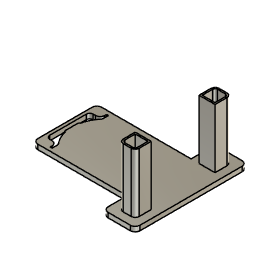
daq_cclamp_3t v2 (Autodesk Fusion 360 design; units mm, degrees)
Autodesk Fusion 360 part; units mm, degrees
sketch "Sketch3" plane through (0, 0, 31.5) normal (0, 0, 1) x (-1, 0, 0)
  arc A0 (-4.334986, -24.725) -> (-4.847966, -25.138298) centre (-4.334986, -25.25) ccw
  line L0 (-4.334986, -24.725) -> (-3.955328, -24.725)
  line L1 (-3.955328, -24.725) -> (-3.955328, -15.275)
  line L2 (-3.955328, -15.275) -> (-4.334986, -15.275)
  arc A1 (-4.847966, -14.861702) -> (-4.334986, -15.275) centre (-4.334986, -14.75) ccw
  arc A2 (-4.847966, -14.861702) -> (-5.656416, -12.00609) centre (-28.445008, -20) ccw
  arc A3 (-5.656416, -12.00609) -> (-9.099786, -6.138625) centre (-23.872376, -18.752159) ccw
  arc A4 (-9.60275, -4.775) -> (-9.099786, -6.138625) centre (-7.50275, -4.775) ccw
  line L3 (-9.60275, -4.775) -> (-9.60275, -1.625)
  line L4 (-9.60275, -1.625) -> (-8.55275, -1.625)
  line L5 (-8.55275, -1.625) -> (-8.55275, -2.675)
  arc A5 (-8.55275, -2.675) -> (-5.40275, -5.825) centre (-5.40275, -2.675) ccw
  line L6 (-5.40275, -5.825) -> (-3.82775, -5.825)
  arc A6 (-1.72775, -7.925) -> (-3.82775, -5.825) centre (-3.82775, -7.925) ccw
  line L7 (-1.72775, -7.925) -> (-1.72775, -32.075)
  arc A7 (-3.82775, -34.175) -> (-1.72775, -32.075) centre (-3.82775, -32.075) ccw
  line L8 (-3.82775, -34.175) -> (-5.40275, -34.175)
  arc A8 (-5.40275, -34.175) -> (-8.55275, -37.325) centre (-5.40275, -37.325) ccw
  line L9 (-8.55275, -37.325) -> (-8.55275, -38.375)
  line L10 (-8.55275, -38.375) -> (-9.60275, -38.375)
  line L11 (-9.60275, -38.375) -> (-9.60275, -35.225)
  arc A9 (-9.099786, -33.861375) -> (-9.60275, -35.225) centre (-7.50275, -35.225) ccw
  arc A10 (-9.099786, -33.861375) -> (-5.656416, -27.99391) centre (-23.872376, -21.247841) ccw
  arc A11 (-5.656416, -27.99391) -> (-4.847966, -25.138298) centre (-28.445008, -20) ccw
  arc A12 (-3, -40) -> (0, -37) centre (-3, -37) ccw
  line L12 (0, -37) -> (0, -3)
  arc A13 (0, -3) -> (-3, 0) centre (-3, -3) ccw
  line L13 (-3, 0) -> (-11, 0)
  line L14 (-11, 0) -> (-11, -40)
  line L15 (-11, -40) -> (-3, -40)
  line L16 (-62, -55) -> (-76, -55)
  line L17 (-79, -52) -> (-79, 12)
  line L18 (-76, 15) -> (-62, 15)
  line L19 (-59, 12) -> (-59, -52)
  line L20 (-11, -40) -> (-59, -40)
  line L21 (-59, -40) -> (-59, 0)
  line L22 (-59, 0) -> (-11, 0)
  line L23 (-11, 0) -> (-11, -40)
  arc A14 (-79, -52) -> (-76, -55) centre (-76, -52) ccw
  arc A15 (-76, 15) -> (-79, 12) centre (-76, 12) ccw
  arc A16 (-59, 12) -> (-62, 15) centre (-62, 12) ccw
  arc A17 (-62, -55) -> (-59, -52) centre (-62, -52) ccw
  arc A18 (-9.054822, -33.201309) -> (-9.533835, -34.5) centre (-7.533835, -34.5) ccw
  arc A19 (-9.130871, -33.136375) -> (-5.869498, -27.57933) centre (-23.123955, -21.18842) ccw
  line L24 (-8.433835, -3.5) -> (-8.433835, -2.4)
  arc A20 (-9.130871, -33.136375) -> (-9.633835, -34.5) centre (-7.533835, -34.5) ccw
  arc A21 (-8.433835, -3.5) -> (-5.533835, -6.4) centre (-5.533835, -3.5) ccw
  arc A22 (-5.717538, -12.54527) -> (-5.775422, -12.386752) centre (-23.123955, -18.81158) ccw
  line L25 (-4.033835, -6.5) -> (-5.533835, -6.5)
  arc A23 (-5.005469, -15.106383) -> (-5.775422, -12.386752) centre (-27.478842, -20) ccw
  line L26 (-9.633835, -2.4) -> (-9.633835, -5.5)
  arc A24 (-5.775422, -27.613248) -> (-5.717538, -27.45473) centre (-23.123955, -21.18842) ccw
  line L27 (-9.533835, -34.5) -> (-9.533835, -37.5)
  arc A25 (-5.533835, -33.5) -> (-8.533835, -36.5) centre (-5.533835, -36.5) ccw
  line L28 (-5.533835, -33.6) -> (-4.033835, -33.6)
  arc A26 (-9.054822, -33.201309) -> (-5.775422, -27.613248) centre (-23.123955, -21.18842) ccw
  arc A27 (-4.516917, -24.4) -> (-5.103179, -24.87234) centre (-4.516917, -25) ccw
  arc A28 (-5.533835, -33.6) -> (-8.433835, -36.5) centre (-5.533835, -36.5) ccw
  arc A29 (-5.005469, -15.106383) -> (-4.516917, -15.5) centre (-4.516917, -15) ccw
  line L29 (-9.533835, -2.5) -> (-9.533835, -5.5)
  arc A30 (-4.033835, -33.6) -> (-1.933835, -31.5) centre (-4.033835, -31.5) ccw
  line L30 (-4.255338, -24.4) -> (-4.516917, -24.4)
  line L31 (-4.516917, -15.5) -> (-4.155338, -15.5)
  arc A31 (-5.775422, -12.386752) -> (-9.054822, -6.798691) centre (-23.123955, -18.81158) ccw
  line L32 (-8.433835, -37.6) -> (-8.433835, -36.5)
  line L33 (-9.633835, -37.6) -> (-8.433835, -37.6)
  arc A32 (-4.516917, -24.5) -> (-5.005469, -24.893617) centre (-4.516917, -25) ccw
  arc A33 (-5.869498, -27.57933) -> (-5.103179, -24.87234) centre (-27.478842, -20) ccw
  arc A34 (-9.533835, -5.5) -> (-9.054822, -6.798691) centre (-7.533835, -5.5) ccw
  line L34 (-5.717538, -27.45473) -> (-5.838432, -27.790548)
  line L35 (-8.433835, -2.4) -> (-9.633835, -2.4)
  arc A35 (-8.533835, -3.5) -> (-5.533835, -6.5) centre (-5.533835, -3.5) ccw
  line L36 (-4.516917, -15.6) -> (-4.255338, -15.6)
  line L37 (-5.838432, -12.209452) -> (-5.717538, -12.54527)
  line L38 (-8.533835, -2.5) -> (-9.533835, -2.5)
  line L39 (-4.155338, -24.5) -> (-4.516917, -24.5)
  line L40 (-9.533835, -37.5) -> (-8.533835, -37.5)
  arc A36 (-2.033835, -8.5) -> (-4.033835, -6.5) centre (-4.033835, -8.5) ccw
  arc A37 (-5.869498, -12.42067) -> (-9.130871, -6.863625) centre (-23.123955, -18.81158) ccw
  arc A38 (-5.775422, -12.386752) -> (-5.838432, -12.209452) centre (-27.478842, -20) ccw
  arc A39 (-5.838432, -27.790548) -> (-5.775422, -27.613248) centre (-27.478842, -20) ccw
  arc A40 (-1.933835, -8.5) -> (-4.033835, -6.4) centre (-4.033835, -8.5) ccw
  line L41 (-0.033835, -40) -> (-0.033835, 0)
  line L42 (-11.033835, 0) -> (-11.033835, -40)
  line L43 (-0.033835, 0) -> (-11.033835, 0)
  line L44 (-11.033835, -40) -> (-0.033835, -40)
  arc A41 (-5.775422, -27.613248) -> (-5.005469, -24.893617) centre (-27.478842, -20) ccw
  line L45 (-4.155338, -15.5) -> (-4.155338, -24.5)
  line L46 (-1.933835, -31.5) -> (-1.933835, -8.5)
  line L47 (-2.033835, -31.5) -> (-2.033835, -8.5)
  line L48 (-4.255338, -15.6) -> (-4.255338, -24.4)
  arc A42 (-4.033835, -33.5) -> (-2.033835, -31.5) centre (-4.033835, -31.5) ccw
  line L49 (-4.033835, -6.4) -> (-5.533835, -6.4)
  line L50 (-8.533835, -3.5) -> (-8.533835, -2.5)
  arc A43 (-5.103179, -15.12766) -> (-4.516917, -15.6) centre (-4.516917, -15) ccw
  line L51 (-5.533835, -33.5) -> (-4.033835, -33.5)
  line L52 (-8.533835, -37.5) -> (-8.533835, -36.5)
  arc A44 (-9.633835, -5.5) -> (-9.130871, -6.863625) centre (-7.533835, -5.5) ccw
  line L53 (-9.633835, -34.5) -> (-9.633835, -37.6)
  arc A45 (-5.103179, -15.12766) -> (-5.869498, -12.42067) centre (-27.478842, -20) ccw
  point P0 (-59, -55)
  point P1 (-79, -55)
  point P2 (-59, 15)
  point P3 (-0.033835, 0)
  point P4 (-1.761584, -20)
  dimension "d17" = 20
  dimension "d18" = 70
  dimension "d19" = 48
  dimension "d20" = 40
  dimension "d21" = 3
  dimension "d61" = 0.1
  dimension "d62" = 11
  dimension "d63" = 40
  constraint horizontal L16
  constraint vertical L17
  constraint horizontal L18
  constraint vertical L19
  constraint horizontal L20
  constraint vertical L21
  constraint horizontal L22
  constraint vertical L23
  constraint coincident L14.end L15.start
  constraint coincident P1 L16
  constraint coincident P1 L17
  constraint tangent L16 A14
  constraint tangent L17 A14
  constraint tangent L17 A15
  constraint tangent L18 A15
  constraint equal A14 A15
  constraint coincident L19 L21
  constraint coincident P2 L18
  constraint coincident P2 L19
  constraint tangent L18 A16
  constraint tangent L19 A16
  constraint equal A14 A16
  constraint coincident P0 L16
  constraint coincident P0 L19
  constraint tangent L16 A17
  constraint tangent L19 A17
  constraint equal A14 A17
  measures "d17" distance of P0 P1
  measures "d18" distance of P0 P2
  measures "d19" distance of L14.end L20.end
  measures "d20" distance of L14.end L13.end
  measures "d21" radius of A14
extrude "Extrude3" add sketch "Sketch3" along normal blind 3 contours A22 L37 A38 | A24 L34 A39 | L9 L10 L11 L33 | A5 L6 A6 L7 A7 L8 A8 A21 L28 A28 A30 A40 L46 L49 | L3 L4 L5 L35 | A12 A13 L13 L14 L15 L23 L41 L43 L44 | A12 L12 A13 L41 | L14 L20 L22 L23 L42 L43 L44 | L19 L20 L21 L22 L42 | L16 L17 L18 L19 L21 A14 A15 A16 A17 picked at (-5.775884, -12.384627) picked at (-5.775884, -27.615373) picked at (-8.90275, -38.116667) picked at (-4.421445, -33.983333) picked at (-9.25275, -1.883333) picked at (-7.788307, -18.375887) picked at (-0.022556, -14.333333) picked at (-11.011278, -26.666667) picked at (-27.022556, -26.666667) picked at (-72.333333, -26.666667) makes body 1 at (42.482617, 24.545325, 34.5) makes body 2 at (5.798134, 12.321391, 33.5) makes body 3 at (5.757836, 27.566669, 33.5)
sketch "Sketch6" plane through (0, 0, 34.5) normal (0, 0, 1) x (-1, 0, 0)
  arc A0 (-79, -52) -> (-76, -55) centre (-76, -52) ccw
  line L0 (-76, -55) -> (-62, -55)
  arc A1 (-62, -55) -> (-59, -52) centre (-62, -52) ccw
  line L1 (-59, -52) -> (-59, -40)
  line L2 (-59, -40) -> (-3, -40)
  arc A2 (-3, -40) -> (0, -37) centre (-3, -37) ccw
  line L3 (0, -37) -> (0, -3)
  arc A3 (0, -3) -> (-3, 0) centre (-3, -3) ccw
  line L4 (-3, 0) -> (-59, 0)
  line L5 (-59, 0) -> (-59, 12)
  arc A4 (-59, 12) -> (-62, 15) centre (-62, 12) ccw
  line L6 (-62, 15) -> (-76, 15)
  arc A5 (-76, 15) -> (-79, 12) centre (-76, 12) ccw
  line L7 (-79, 12) -> (-79, -52)
  line L8 (-66.5, -50) -> (-71.5, -50)
  line L9 (-74, -47.5) -> (-74, -40)
  line L10 (-74, -40) -> (-64, -40)
  line L11 (-64, -40) -> (-64, -47.5)
  line L12 (-64, 0) -> (-74, 0)
  line L13 (-74, 0) -> (-74, 7.5)
  line L14 (-71.5, 10) -> (-66.5, 10)
  line L15 (-64, 7.5) -> (-64, 0)
  arc A6 (-66.5, -50) -> (-64, -47.5) centre (-66.5, -47.5) ccw
  arc A7 (-74, -47.5) -> (-71.5, -50) centre (-71.5, -47.5) ccw
  arc A8 (-71.5, 10) -> (-74, 7.5) centre (-71.5, 7.5) ccw
  arc A9 (-64, 7.5) -> (-66.5, 10) centre (-66.5, 7.5) ccw
  line L16 (-4.255338, -15.6) -> (-4.516917, -15.6)
  arc A10 (-5.103179, -15.12766) -> (-4.516917, -15.6) centre (-4.516917, -15) ccw
  arc A11 (-5.103179, -15.12766) -> (-5.869498, -12.42067) centre (-27.478842, -20) ccw
  arc A12 (-5.869498, -12.42067) -> (-9.130871, -6.863625) centre (-23.123955, -18.81158) ccw
  arc A13 (-9.633835, -5.5) -> (-9.130871, -6.863625) centre (-7.533835, -5.5) ccw
  line L17 (-9.633835, -5.5) -> (-9.633835, -2.4)
  line L18 (-9.633835, -2.4) -> (-8.433835, -2.4)
  line L19 (-8.433835, -2.4) -> (-8.433835, -3.5)
  arc A14 (-8.433835, -3.5) -> (-5.533835, -6.4) centre (-5.533835, -3.5) ccw
  line L20 (-5.533835, -6.4) -> (-4.033835, -6.4)
  arc A15 (-1.933835, -8.5) -> (-4.033835, -6.4) centre (-4.033835, -8.5) ccw
  line L21 (-1.933835, -8.5) -> (-1.933835, -31.5)
  arc A16 (-4.033835, -33.6) -> (-1.933835, -31.5) centre (-4.033835, -31.5) ccw
  line L22 (-4.033835, -33.6) -> (-5.533835, -33.6)
  arc A17 (-5.533835, -33.6) -> (-8.433835, -36.5) centre (-5.533835, -36.5) ccw
  line L23 (-8.433835, -36.5) -> (-8.433835, -37.6)
  line L24 (-8.433835, -37.6) -> (-9.633835, -37.6)
  line L25 (-9.633835, -37.6) -> (-9.633835, -34.5)
  arc A18 (-9.130871, -33.136375) -> (-9.633835, -34.5) centre (-7.533835, -34.5) ccw
  arc A19 (-9.130871, -33.136375) -> (-5.869498, -27.57933) centre (-23.123955, -21.18842) ccw
  arc A20 (-5.869498, -27.57933) -> (-5.103179, -24.87234) centre (-27.478842, -20) ccw
  arc A21 (-4.516917, -24.4) -> (-5.103179, -24.87234) centre (-4.516917, -25) ccw
  line L26 (-4.516917, -24.4) -> (-4.255338, -24.4)
  line L27 (-4.255338, -24.4) -> (-4.255338, -15.6)
  point P0 (-64, -50)
  point P1 (-74, -50)
  point P2 (-64, 10)
  dimension "d36" = 10
  dimension "d37" = 10
  dimension "d38" = 10
  dimension "d39" = 10
  dimension "d40" = 5
  dimension "d41" = 5
  dimension "d42" = 5
  dimension "d43" = 5
  dimension "d44" = 2.5
  constraint horizontal L8
  constraint vertical L9
  constraint horizontal L10
  constraint vertical L11
  constraint horizontal L12
  constraint vertical L13
  constraint horizontal L14
  constraint vertical L15
  constraint coincident P0 L8
  constraint coincident P0 L11
  constraint tangent L8 A6
  constraint tangent L11 A6
  constraint coincident P1 L8
  constraint coincident P1 L9
  constraint tangent L8 A7
  constraint tangent L9 A7
  constraint equal A6 A7
  constraint tangent L13 A8
  constraint tangent L14 A8
  constraint equal A6 A8
  constraint coincident P2 L14
  constraint coincident P2 L15
  constraint tangent L14 A9
  constraint tangent L15 A9
  constraint equal A6 A9
  measures "d36" distance of P0 P1
  measures "d37" distance of P0 L10.end
  measures "d38" distance of L12.start L12.end
  measures "d39" distance of L12.start P2
  measures "d40" distance of L0 L8
  measures "d41" distance of L6 L14
  measures "d42" distance of L7 L9
  measures "d43" distance of L5 L15
  measures "d44" radius of A6
extrude "Extrude6" add sketch "Sketch6" along normal blind 37 thin wall 1 inside contours L8 L9 L10 L11 A6 A7 | L12 L13 L14 L15 A8 A9 picked at (-70.666667, -42.5) picked at (-67.333333, 5) bodies 1
